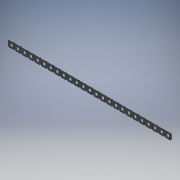
# Autodesk Inventor part: Bar 1x20
Saved by Autodesk Inventor 2018 (Build 220112000, 112)
## iProperties
Category: Structure
Company: Autodesk Inc.
Created: 2012-03-24
Part Number: Bar 1x20
Document SubType Name: Sheet Metal
Density: 7.85 g/cm^3
Mass: 26.4956 g
Surface Area: 65.1076 cm^2
Volume: 3.37523 cm^3
Sheet Metal Rule: Default
Material: Steel
Catalog Web Link: http://www.vexrobotics.com/products/accessories/structure/275-1141.html
Vendor: VEX
Appearance: Zinc
Author: Autodesk Inc.
Autodesk Inventor part; units mm, degrees
ref_plane "YZ Plane" through (0, 0, 0) normal (1, 0, 0) x (0, 1, 0)
ref_plane "XZ Plane" through (0, 0, 0) normal (0, 1, 0) x (-1, 0, 0)
ref_plane "XY Plane" through (0, 0, 0) normal (0, 0, 1) x (1, 0, 0)
sketch "Sketch1" plane through (0, 0, 0) normal (0, 0, 1) x (1, 0, 0)
  line L0 (-15.0193, 9.7889) -> (-23.9093, 9.7889)
  line L1 (-25.8143, 7.8839) -> (-25.8143, -1.0061)
  line L2 (-23.9093, -2.9111) -> (-15.0193, -2.9111)
  line L3 (-13.1143, -1.0061) -> (-13.1143, 7.8839)
  line L4 (-25.8143, 7.8839) -> (-23.9093, 9.7889)
  line L5 (-25.8143, -1.0061) -> (-23.9093, -2.9111)
  line L6 (-15.0193, -2.9111) -> (-13.1143, -1.0061)
  line L7 (-13.1143, 7.8839) -> (-15.0193, 9.7889)
  line L8 (-21.2931, 5.7249) -> (-17.6863, 5.7249)
  line L9 (-17.1783, 5.2169) -> (-17.1783, 1.6101)
  line L10 (-17.6863, 1.1021) -> (-21.2931, 1.1021)
  line L11 (-21.8011, 1.6101) -> (-21.8011, 5.2169)
  arc A0 (-21.2931, 5.7249) -> (-21.8011, 5.2169) centre (-21.2931, 5.2169) ccw
  arc A1 (-17.1783, 5.2169) -> (-17.6863, 5.7249) centre (-17.6863, 5.2169) ccw
  arc A2 (-17.6863, 1.1021) -> (-17.1783, 1.6101) centre (-17.6863, 1.6101) ccw
  arc A3 (-21.8011, 1.6101) -> (-21.2931, 1.1021) centre (-21.2931, 1.6101) ccw
  point P0 (-13.1143, 9.7889)
  point P1 (-25.8143, -2.9111)
  point P2 (-25.8143, 9.7889)
  point P3 (-13.1143, -2.9111)
  point P4 (-21.8011, 5.7249)
  point P5 (-17.1783, 1.1021)
  point P6 (-17.1783, 5.7249)
  point P7 (-21.8011, 1.1021)
  dimension "d0" = 12.7
  dimension "d1" = 12.7
  dimension "d2" = 1.905
  dimension "d3" = 1.905
  dimension "d4" = 1.905
  dimension "d5" = 1.905
  dimension "d6" = 1.905
  dimension "d7" = 1.905
  dimension "d8" = 1.905
  dimension "d9" = 1.905
  dimension "d10" = 4.6228
  dimension "d11" = 4.6228
  dimension "d12" = 4.064
  dimension "d13" = 4.064
  dimension "d18" = 0.508
  measures "d0" distance of point (-25.814, 9.789) point (-25.814, -2.911)
  measures "d1" distance of point (-13.114, 9.789) point (-25.814, 9.789)
  measures "d2" distance of L1.start point (-25.814, 9.789)
  measures "d3" distance of L0.end point (-25.814, 9.789)
  measures "d4" distance of L1.end point (-25.814, -2.911)
  measures "d5" distance of L2.start point (-25.814, -2.911)
  measures "d6" distance of L2.end point (-13.114, -2.911)
  measures "d7" distance of L3.start point (-13.114, -2.911)
  measures "d8" distance of L3.end point (-13.114, 9.789)
  measures "d9" distance of L0.start point (-13.114, 9.789)
  measures "d10" distance of point (-21.801, 1.102) point (-21.801, 5.725)
  measures "d11" distance of point (-17.178, 1.102) point (-21.801, 1.102)
  measures "d12" distance between parallel lines of L0 L8
  measures "d13" distance between parallel lines of L3 L9
  measures "d18" radius of A0
extrude "Plate1" add sketch "Sketch1" along normal blind 1.27
pattern_linear "Rectangular Pattern1" count 25 spacing 12.7 along (1, 0, 0)
sketch "Sketch4" plane through (-23.9093, 9.7889, 1.27) normal (0, 0, 1) x (1, 0, 0)
  line L0 (6.731, -4.572) -> (6.731, -8.1788) projected
  line L1 (6.223, -8.6868) -> (2.6162, -8.6868) projected
  line L2 (2.6162, -4.064) -> (6.223, -4.064) projected
  circle A0 centre (4.4196, -6.3754) radius 2.3114
  point P0 (23.9093, -9.7889)
  constraints: 3 tangent, 1 centre point
surface extrude "ExtrusionSrf1" sketch "Sketch4" against normal up to surface (1.27 mm away) shown no curves A0
pattern_linear "Rectangular Pattern2" count 25 spacing 12.7 along (1, 0, 0) of "ExtrusionSrf1"
equation "\"d64\" = Thickness"
equation "\"d3\" = d2"
equation "\"d4\" = d2"
equation "\"d5\" = d4"
equation "\"d6\" = d2"
equation "\"d7\" = d6"
equation "\"d8\" = d2"
equation "\"d9\" = d8"
equation "\"BendRadius\" = Thickness"
equation "\"BendReliefWidth\" = Thickness"
equation "\"BendReliefDepth\" = 0.5 * Thickness"
equation "\"CornerReliefSize\" = 4 * Thickness"
equation "\"MinimumRemnant\" = 2 * Thickness"
equation "\"TransitionRadius\" = BendRadius"
equation "\"d14\" = BendRadius"
equation "\"JacobiRadiusSize\" = Thickness"
equation "\"GapSize\" = Thickness"
equation "\"Thickness\" = 1.27"
body "Solid1"
body "Srf1"
body "Srf2"
body "Srf3"
body "Srf4"
body "Srf5"
body "Srf6"
body "Srf7"
body "Srf8"
body "Srf9"
body "Srf10"
body "Srf11"
body "Srf12"
body "Srf13"
body "Srf14"
body "Srf15"
body "Srf16"
body "Srf17"
body "Srf18"
body "Srf19"
body "Srf20"
body "Srf21"
body "Srf22"
body "Srf23"
body "Srf24"
body "Srf25"
